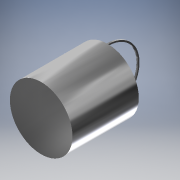
# Autodesk Inventor part: emmer
Saved by Autodesk Inventor 2017 (Build 210142000, 142)
## iProperties
Created: 2017-02-19
Part Number: emmer
Material: Generic
Document SubType Name: Modeling
Designer: user
Density: 1 g/cm^3
Appearance: Honed
Author: user
Autodesk Inventor part; units mm, degrees
ref_plane "YZ Plane" through (0, 0, 0) normal (1, 0, 0) x (0, 1, 0)
ref_plane "XZ Plane" through (0, 0, 0) normal (0, 1, 0) x (-1, 0, 0)
ref_plane "XY Plane" through (0, 0, 0) normal (0, 0, 1) x (1, 0, 0)
sketch "Sketch1" plane through (0, 0, 0) normal (0, 1, 0) x (-1, 0, 0)
  circle A0 centre (0, 0) radius 85
  dimension "d0" = 170
  constraints: 1 centre point, 1 coincident
  measures "d0" diameter of A0
extrude "Extrusion1" add sketch "Sketch1" along normal blind 180
shell "Shell1" thickness 2 removed faces 1 at (4.1372, 180, 51.3099)
sketch "Sketch2" plane through (0, 0, 0) normal (1, 0, 0) x (0, 1, 0)
  line L0 (180, -85) -> (180, 85) projected
  line L1 (0, 85) -> (0, -85) projected
  arc A0 (180, -85) -> (180, 85) centre (180, 0) ccw
  line L2 (0, 85) -> (180, 85) projected
  line L3 (0, -85) -> (180, -85) projected
  arc A1 (180, -81) -> (180, 81) centre (180, 0) ccw
  point P0 (0, 0)
  dimension "d4" = 4
  constraints: 4 point on circle, 2 centre point, 2 point on line, 1 tangent
  measures "d4" radial gap between concentric circles of A0 A1
extrude "Extrusion2" add sketch "Sketch2" along normal mid plane 4 contours L0 A1 A0
body "Solid1"
